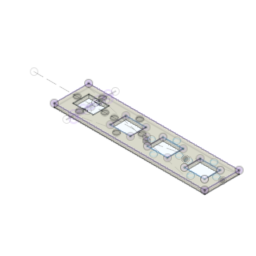
Buttons_Final (Autodesk Fusion 360 design; units mm, degrees)
Autodesk Fusion 360 part; units mm, degrees
note: some values were not read from the file. Chosen so that the rebuilt part matches the saved one: which face or edge a step refers to. Set by a fixed rule: which sketch regions a step uses.
(part 1 of 4)
sketch "Sketch1" plane through (0, 0, 0) normal (0, 1, 0) x (1, 0, 0) in component "Box"
  line L0 (86.75, -29) -> (-86.75, -29)
  line L1 (-86.75, -29) -> (-86.75, 29)
  line L2 (-86.75, 29) -> (86.75, 29)
  line L3 (86.75, 29) -> (86.75, -29)
  line L4 (86.75, -29) -> (-86.75, 29) construction
  line L5 (-86.75, -29) -> (86.75, 29) construction
  dimension "d407" = 173.5
  dimension "d408" = 58
  dimension "d1076" = 0
  dimension "d1077" = 0
  dimension "d1078" = 0
  dimension "d1079" = 0
  dimension "d1179" = 0
  dimension "d1180" = 0
  dimension "d1181" = 0
  dimension "d1182" = 0
  dimension "d1239" = 0
  dimension "d1240" = 0
  dimension "d1241" = 0
  dimension "d1242" = 0
  dimension "d1263" = 0
  dimension "d1264" = 0
  dimension "d1265" = 0
  dimension "d1266" = 0
  dimension "d1515" = 0
  dimension "d1516" = 0
  dimension "d1517" = 0
  dimension "d1518" = 0
  constraint perpendicular L0 L1
  constraint parallel L0 L2
  constraint parallel L1 L3
  constraint horizontal L0
  constraint coincident L4 origin
  constraint coincident L5 origin
  measures "d407" distance of L1.end L2.end
  measures "d408" distance of L0.end L1.end
extrude "Extrude1" add sketch "Sketch1" along normal blind 33 makes body 1 in component "Box"
sketch "Sketch2" plane through (0, 33, 0) normal (0, 1, 0) x (-1, 0, 0) in component "Box"
  line L0 (-86.75, -29) -> (86.75, -29)
  line L1 (86.75, -29) -> (86.75, 29)
  line L2 (86.75, 29) -> (-86.75, 29)
  line L3 (-86.75, 29) -> (-86.75, -29)
  line L4 (83.75, 26) -> (-83.75, 26)
  line L5 (-83.75, 26) -> (-83.75, -26)
  line L6 (-83.75, -26) -> (83.75, -26)
  line L7 (83.75, -26) -> (83.75, 26)
  dimension "d569" = -3
extrude "Extrude2" cut sketch "Sketch2" against normal up to surface (30 mm away) contours L4 L5 L6 L7 bodies 1 in component "Box"
sketch "Sketch5" plane through (0, 0, 29) normal (0, 0, 1) x (1, 0, 0) in component "Box"
  line L0 (-86.75, 0) -> (86.75, 0)
  line L1 (86.75, 0) -> (86.75, 33)
  line L2 (86.75, 33) -> (-86.75, 33)
  line L3 (-86.75, 33) -> (-86.75, 0)
  line L4 (-83.75, 3) -> (83.75, 3)
  line L5 (83.75, 3) -> (83.75, 33)
  line L6 (-83.75, 33) -> (-83.75, 3)
  line L7 (-47, 33) -> (83.75, 33)
  line L8 (86.75, 23) -> (86.75, 33)
  line L9 (83.75, 33) -> (86.75, 33)
  line L10 (-86.75, 33) -> (-83.75, 33)
  dimension "d440" = 3
  dimension "d441" = 3
  dimension "d442" = 3
  dimension "d595" = 10
  constraint coincident L2 L7.start
  constraint coincident L2 L5.end
  constraint parallel L0 L4
  constraint parallel L1 L5
  constraint parallel L3 L6
  constraint coincident L2 L6.start
  constraint coincident L1.end L2.start
  constraint coincident L1 L8.start
  constraint coincident L2.end L3.start
  measures "d440" distance of L0 L4
  measures "d441" distance of L3 L6
  measures "d442" distance of L1 L5
  measures "d595" distance of L1.end L8.start
extrude "Extrude5" cut sketch "Sketch5" against normal up to surface (3 mm away) contours L2 L4 L5 L6 L7 bodies 1 in component "Box"
sketch "Sketch3" plane through (0, 0, 29) normal (0, 0, 1) x (1, 0, 0) in component "Box"
  line L0 (-86.75, 0) -> (86.75, 0)
  line L1 (86.75, 0) -> (86.75, 33)
  line L2 (-86.75, 33) -> (-86.75, 0)
  line L3 (-86.75, 33) -> (-83.75, 33)
  line L4 (73.75, 21) -> (83.75, 21)
  line L5 (73.75, 21) -> (73.75, 3)
  line L6 (73.75, 3) -> (83.75, 3)
  line L7 (83.75, 3) -> (83.75, 21)
  line L8 (86.75, 0) -> (-86.75, 0)
  line L9 (-83.75, 33) -> (83.75, 33)
  line L10 (-83.75, 21) -> (-73.75, 21)
  line L11 (-73.75, 21) -> (-73.75, 3)
  line L12 (-73.75, 3) -> (-83.75, 3)
  line L13 (-83.75, 3) -> (-83.75, 21)
  line L14 (83.75, 33) -> (83.75, 3)
  line L15 (83.75, 3) -> (-83.75, 3)
  line L16 (-83.75, 3) -> (-83.75, 33)
  line L17 (86.75, 33) -> (83.75, 33)
  line L18 (83.75, 33) -> (86.75, 33)
  point P0 (0, 16.5)
  dimension "d424" = 10
  dimension "d1313" = 3
  dimension "d1315" = 12
  dimension "d1316" = 3
  dimension "d1566" = 10
  dimension "d1568" = 12
  dimension "d1570" = 3
  dimension "d1571" = 3
  constraint perpendicular L4 L5
  constraint perpendicular L5 L6
  constraint horizontal L10
  constraint vertical L11
  constraint horizontal L12
  constraint vertical L13
  measures "d424" distance of L4.end L4.start
  measures "d1313" distance of L6 L8
  measures "d1315" distance of L4 L9
  measures "d1316" distance of L1 L7
  measures "d1566" distance of L10.start L10.end
  measures "d1568" distance of L9 L10
  measures "d1570" distance of L8 L12
  measures "d1571" distance of L2 L13
extrude "Extrude3" add sketch "Sketch3" along normal mid plane 10 from surface at -45 contours L4 L5 L6 L7 L14 L15 bodies 1 in component "Box"
mirror "Mirror1" about plane through (0, 0, 0) normal (0, 0, 1) of "Extrude3" in component "Box"
sketch "Sketch4" plane through (0, 33, 0) normal (0, 1, 0) x (-1, 0, 0) in component "Box"
  line L0 (-86.75, -29) -> (86.75, -29)
  line L1 (86.75, -29) -> (86.75, 29)
  line L2 (-83.75, 29) -> (-86.75, 29)
  line L3 (-86.75, 29) -> (-86.75, -29)
  circle A0 centre (79.75, -24.8) radius 2
  line L4 (83.75, -26) -> (-83.75, -26)
  line L5 (-83.75, -26) -> (-83.75, 29)
  circle A1 centre (79.75, 24.8) radius 2
  line L6 (86.75, 29) -> (86.75, -29)
  line L7 (86.75, 29) -> (73.75, 29)
  line L8 (73.75, 29) -> (73.75, 21)
  line L9 (73.75, 21) -> (86.75, 21)
  line L10 (86.75, 21) -> (86.75, 29)
  line L11 (86.75, -29) -> (73.75, -29)
  line L12 (73.75, -29) -> (73.75, -21)
  line L13 (73.75, -21) -> (86.75, -21)
  line L14 (86.75, -21) -> (86.75, -29)
  line L15 (86.75, 29) -> (83.75, 29)
  dimension "d431" = 4
  dimension "d581" = 4.2
  dimension "d586" = 4
  dimension "d587" = 4.2
  dimension "d933" = 0
  dimension "d934" = 0
  dimension "d935" = 0
  dimension "d933_1" = 0
  dimension "d934_1" = 0
  dimension "d935_1" = 0
  dimension "d933_2" = 0
  dimension "d934_2" = 0
  dimension "d935_2" = 0
  dimension "d1672" = 7
  dimension "d1673" = 13
  dimension "d1674" = 8
  dimension "d1675" = 8
  dimension "d1676" = 13
  dimension "d1677" = 7
  constraint horizontal L7
  constraint vertical L8
  constraint horizontal L9
  constraint vertical L10
  constraint coincident L1.end L6.start
  constraint horizontal L11
  constraint vertical L12
  constraint horizontal L13
  constraint vertical L14
  constraint coincident L0.end L1.start
  measures "d431" diameter of A0
  measures "d581" distance of L0 A0.centre
  measures "d586" diameter of A1
  measures "d587" distance of L2 A1.centre
  measures "d1672" distance of A1.centre L6
  measures "d1673" distance of L1.end L7.end
  measures "d1674" distance of L1.end L9.end
  measures "d1675" distance of L0.end L13.end
  measures "d1676" distance of L0.end L11.end
  measures "d1677" distance of A0.centre L14
extrude "Extrude4" add sketch "Sketch4" against normal up to surface (30 mm away) contours L0 L1 L6 L11 L12 L13 L14 | L1 L6 L7 L8 L9 L10 L15 | A0 L4 | A0 L4 bodies 1 in component "Box"
mirror "Mirror2" about plane through (0, 0, 0) normal (1, 0, 0) of "Extrude4" in component "Box"
sketch "Sketch7" plane through (0, 33, 0) normal (0, 1, 0) x (-1, 0, 0) in component "Box"
  circle A0 centre (79.75, -24.8) radius 2
  line L0 (73.75, -26) -> (-73.75, -26)
  line L1 (-73.75, 29) -> (-86.75, 29)
  line L2 (-86.75, 29) -> (-86.75, -29)
  line L3 (-86.75, -29) -> (86.75, -29)
  line L4 (86.75, -29) -> (86.75, 29)
  line L5 (-73.75, 29) -> (73.75, 29)
  line L6 (86.75, 29) -> (86.75, -29)
  line L7 (-83.75, -21) -> (-83.75, 21)
  line L8 (73.75, 29) -> (73.75, 21)
  line L9 (73.75, 21) -> (83.75, 21)
  line L10 (83.75, 21) -> (83.75, -21)
  line L11 (83.75, -21) -> (73.75, -21)
  line L12 (73.75, -21) -> (73.75, -26)
  line L13 (-73.75, -26) -> (-73.75, -21)
  line L14 (-73.75, -21) -> (-83.75, -21)
  line L15 (-83.75, 21) -> (-73.75, 21)
  line L16 (-73.75, 21) -> (-73.75, 29)
  line L17 (86.75, 29) -> (73.75, 29)
  circle A1 centre (-79.75, 24.8) radius 2
  line L18 (86.75, -21) -> (86.75, -29)
  point P0 (87, 25)
  point P1 (79.75, -24.8)
  dimension "d570" = 4
  dimension "d584" = 4.2
  dimension "d1679" = 7
  measures "d570" diameter of A0
  measures "d584" distance of A0.centre L3
  measures "d1679" distance of A0.centre L18
sketch "Sketch1 (2)" plane through (0, 33, 0) normal (0, 1, 0) x (-1, 0, 0) in component "Lid"
  line L0 (-73.75, 29) -> (-86.75, 29)
  line L1 (-86.75, 29) -> (-86.75, -29)
  line L2 (-86.75, -29) -> (86.75, -29)
  line L3 (86.75, -29) -> (86.75, 29)
  line L4 (73.75, -26) -> (-73.75, -26)
  line L5 (73.75, -26) -> (-73.75, -26)
  line L6 (-83.75, 11) -> (-83.75, -11)
  line L7 (-73.75, -26) -> (73.75, -26)
  line L8 (83.75, -21) -> (83.75, 21)
  line L9 (73.75, 29) -> (-73.75, 29)
  line L10 (86.75, -29) -> (93.75, -29)
  line L11 (93.75, -29) -> (93.75, 32)
  line L12 (93.75, 32) -> (-93.75, 32)
  line L13 (-93.75, 32) -> (-93.75, -29)
  line L14 (-93.75, -29) -> (86.75, -29)
  line L15 (-93.75, 29) -> (93.75, 29)
  line L16 (93.75, 29) -> (93.75, -29)
  line L17 (93.75, -29) -> (-93.75, -29)
  line L18 (-93.75, -29) -> (-93.75, 29)
  line L19 (-93.75, 29) -> (93.75, -29) construction
  line L20 (93.75, 29) -> (-93.75, -29) construction
  line L21 (-73.75, 29) -> (-73.75, 11)
  line L22 (-73.75, 11) -> (-83.75, 11)
  line L23 (-83.75, -11) -> (-73.75, -11)
  line L24 (-73.75, -11) -> (-73.75, -26)
  line L25 (-83.75, -21) -> (-83.75, 21)
  line L26 (73.75, 29) -> (73.75, 21)
  line L27 (73.75, 21) -> (83.75, 21)
  line L28 (83.75, 21) -> (83.75, -21)
  line L29 (83.75, -21) -> (73.75, -21)
  line L30 (73.75, -21) -> (73.75, -26)
  line L31 (-73.75, -26) -> (-73.75, -21)
  line L32 (-73.75, -21) -> (-83.75, -21)
  line L33 (-83.75, 21) -> (-73.75, 21)
  line L34 (-73.75, 21) -> (-73.75, 29)
  line L35 (86.75, 29) -> (73.75, 29)
  line L36 (73.75, -26) -> (73.75, -21)
  line L37 (73.75, -21) -> (83.75, -21)
  line L38 (83.75, 21) -> (73.75, 21)
  line L39 (73.75, 21) -> (73.75, 29)
  circle A0 centre (-79.75, 24.8) radius 2
  circle A1 centre (79.75, 24.8) radius 2
  dimension "d1017" = 3
  dimension "d1018" = 10
  dimension "d1020" = 187.5
  dimension "d1072" = 0
  dimension "d1073" = 0
  dimension "d1074" = 0
  dimension "d1075" = 0
  dimension "d1235" = 0
  dimension "d1236" = 0
  dimension "d1237" = 0
  dimension "d1238" = 0
  dimension "d1449" = 0
  dimension "d1450" = 0
  dimension "d1451" = 0
  dimension "d1452" = 0
  dimension "d1463" = 0
  dimension "d1464" = 0
  dimension "d1465" = 0
  dimension "d1466" = 0
  dimension "d1495" = 0
  dimension "d1496" = 0
  dimension "d1497" = 0
  dimension "d1498" = 0
  dimension "d1507" = 0
  dimension "d1508" = 0
  dimension "d1509" = 0
  dimension "d1510" = 0
  dimension "d1511" = 0
  dimension "d1512" = 0
  dimension "d1513" = 0
  dimension "d1514" = 0
  dimension "d1531" = 0
  dimension "d1532" = 0
  dimension "d1533" = 0
  dimension "d1534" = 0
  constraint coincident L2.end L3.start
  constraint perpendicular L3 L10
  constraint perpendicular L10 L11
  constraint perpendicular L11 L12
  constraint perpendicular L12 L13
  constraint perpendicular L3 L14
  constraint perpendicular L15 L16
  constraint parallel L15 L17
  constraint parallel L16 L18
  constraint horizontal L15
  constraint coincident L13 L15.start
  constraint coincident L19 origin
  constraint coincident L20 origin
  measures "d1017" distance of L9 L12
  measures "d1018" distance of L8 L11
  measures "d1020" distance of L11.end L12.end
extrude "Extrude2'" add sketch "Sketch1 (2)" along normal blind 5.25 separate body contours L0 L1 L2 L3 L4 L5 L6 L7 L8 L14 L15 L17 L21 L24 L25 L26 L27 L28 L29 L30 L31 L32 L33 L34 L35 L36 L37 L38 L39 | L4 L5 L6 L7 L8 L9 L15 L21 L22 L23 L24 L25 L26 L27 L28 L29 L30 L31 L34 L36 L37 L38 L39 | L1 L13 L14 L15 L17 L18 | L21 L22 L25 L33 | L3 L10 L11 L15 L16 L17 | L23 L24 L25 L32 | A0 | A1 makes body 2 in component "Lid"
sketch "Sketch1 (3)" plane through (0, 3, 0) normal (0, 1, 0) x (-1, 0, 0) in component "Button Base"
  line L0 (-83.5, 19.1) -> (83.5, 19.1)
  line L1 (83.5, 19.1) -> (83.5, -19.1)
  line L2 (83.5, -19.1) -> (-83.5, -19.1)
  line L3 (-83.5, -19.1) -> (-83.5, 19.1)
  line L4 (-83.5, 19.1) -> (83.5, -19.1) construction
  line L5 (83.5, 19.1) -> (-83.5, -19.1) construction
  dimension "d738" = 167
  dimension "d739" = 38.2
  dimension "d917" = 0
  dimension "d918" = 0
  dimension "d919" = 0
  dimension "d920" = 0
  dimension "d943" = 0
  dimension "d944" = 0
  dimension "d945" = 0
  dimension "d946" = 0
  dimension "d955" = 0
  dimension "d956" = 0
  dimension "d957" = 0
  dimension "d958" = 0
  dimension "d963" = 0
  dimension "d964" = 0
  dimension "d965" = 0
  dimension "d966" = 0
  dimension "d973" = 0
  dimension "d974" = 0
  dimension "d975" = 0
  dimension "d976" = 0
  dimension "d985" = 0
  dimension "d986" = 0
  dimension "d987" = 0
  dimension "d988" = 0
  dimension "d1007" = 0
  dimension "d1008" = 0
  dimension "d1009" = 0
  dimension "d1010" = 0
  dimension "d1090" = 0
  dimension "d1091" = 0
  dimension "d1092" = 0
  dimension "d1093" = 0
  dimension "d1098" = 0
  dimension "d1099" = 0
  dimension "d1100" = 0
  dimension "d1101" = 0
  dimension "d1107" = 0
  dimension "d1108" = 0
  dimension "d1109" = 0
  dimension "d1110" = 0
  dimension "d1115" = 0
  dimension "d1116" = 0
  dimension "d1117" = 0
  dimension "d1118" = 0
  dimension "d1123" = 0
  dimension "d1124" = 0
  dimension "d1125" = 0
  dimension "d1126" = 0
  dimension "d1132" = 0
  dimension "d1133" = 0
  dimension "d1134" = 0
  dimension "d1135" = 0
  dimension "d1140" = 0
  dimension "d1141" = 0
  dimension "d1142" = 0
  dimension "d1143" = 0
  dimension "d1148" = 0
  dimension "d1149" = 0
  dimension "d1150" = 0
  dimension "d1151" = 0
  dimension "d1160" = 0
  dimension "d1161" = 0
  dimension "d1162" = 0
  dimension "d1163" = 0
  dimension "d1175" = 0
  dimension "d1176" = 0
  dimension "d1177" = 0
  dimension "d1178" = 0
  dimension "d1191" = 0
  dimension "d1192" = 0
  dimension "d1193" = 0
  dimension "d1194" = 0
  dimension "d1199" = 0
  dimension "d1200" = 0
  dimension "d1201" = 0
  dimension "d1202" = 0
  dimension "d1215" = 0
  dimension "d1216" = 0
  dimension "d1217" = 0
  dimension "d1218" = 0
  dimension "d1247" = 0
  dimension "d1248" = 0
  dimension "d1249" = 0
  dimension "d1250" = 0
  dimension "d1255" = 0
  dimension "d1256" = 0
  dimension "d1257" = 0
  dimension "d1258" = 0
  dimension "d1259" = 0
  dimension "d1260" = 0
  dimension "d1261" = 0
  dimension "d1262" = 0
  dimension "d1279" = 0
  dimension "d1280" = 0
  dimension "d1281" = 0
  dimension "d1282" = 0
  dimension "d1287" = 0
  dimension "d1288" = 0
  dimension "d1289" = 0
  dimension "d1290" = 0
  constraint perpendicular L0 L1
  constraint parallel L0 L2
  constraint parallel L1 L3
  constraint horizontal L0
  constraint coincident L4 origin
  constraint coincident L5 origin
  measures "d738" distance of L1.end L2.end
  measures "d739" distance of L0.end L1.end
extrude "Extrude1'" add sketch "Sketch1 (3)" along normal blind 4 separate body makes body 3 in component "Button Base"
sketch "Sketch2 (2)" plane through (0, 7, 0) normal (0, 1, 0) x (-1, 0, 0) in component "Button Base"
  line L0 (73, -8.7) -> (50.6, -8.7)
  line L1 (50.6, -8.7) -> (50.6, 8.7)
  line L2 (50.6, 8.7) -> (73, 8.7)
  line L3 (73, 8.7) -> (73, -8.7)
  line L4 (0, 0) -> (125, 0) construction
  line L5 (9.4, -8.7) -> (9.4, 8.7)
  line L6 (31.8, -8.7) -> (9.4, -8.7)
  line L7 (31.8, 8.7) -> (31.8, -8.7)
  line L8 (9.4, 8.7) -> (31.8, 8.7)
  line L9 (-31.8, -8.7) -> (-31.8, 8.7)
  line L10 (-9.4, -8.7) -> (-31.8, -8.7)
  line L11 (-9.4, 8.7) -> (-9.4, -8.7)
  line L12 (-31.8, 8.7) -> (-9.4, 8.7)
  line L13 (-73, -8.7) -> (-73, 8.7)
  line L14 (-50.6, 8.7) -> (-50.6, -8.7)
  line L15 (-50.6, -8.7) -> (-73, -8.7)
  line L16 (-73, 8.7) -> (-50.6, 8.7)
  line L17 (-83.5, -19.1) -> (83.5, -19.1)
  line L18 (83.5, -19.1) -> (83.5, 19.1)
  line L19 (83.5, 19.1) -> (-83.5, 19.1)
  line L20 (-83.5, 19.1) -> (-83.5, -19.1)
  point P0 (-43, 0)
  point P1 (-43, 0)
  point P2 (-84, 0)
  point P3 (-84, 0)
  point P4 (-123, 0)
  point P5 (-123, 0)
  dimension "d460" = 22.4
  dimension "d461" = 17.4
  dimension "d462" = 8.7
  dimension "d684" = 22.4
  dimension "d685" = 17.4
  dimension "d686" = 18.8
  dimension "d687" = 22.4
  dimension "d688" = 17.4
  dimension "d689" = 18.8
  dimension "d690" = 22.4
  dimension "d691" = 17.4
  dimension "d692" = 18.8
  dimension "d741" = 10.5
  dimension "d742" = 9.5
  constraint horizontal L0
  constraint vertical L1
  constraint horizontal L2
  constraint vertical L3
  constraint coincident L4.start origin
  constraint horizontal L6
  constraint vertical L5
  constraint horizontal L8
  constraint vertical L7
  constraint coincident P1 P0
  constraint horizontal L10
  constraint vertical L9
  constraint horizontal L12
  constraint vertical L11
  constraint coincident P3 P2
  constraint horizontal L15
  constraint vertical L13
  constraint horizontal L16
  constraint vertical L14
  constraint coincident P5 P4
  measures "d460" distance of L0.start L0.end
  measures "d461" distance of L0.start L2.end
  measures "d462" distance of L0 L4
  measures "d684" distance of L5.start L6.start
  measures "d685" distance of L7.start L6.start
  measures "d686" distance of L1 L7
  measures "d687" distance of L10.start L9.start
  measures "d688" distance of L10.start L11.start
  measures "d689" distance of L5 L11
  measures "d690" distance of L13.start L14.end
  measures "d691" distance of L14.start L14.end
  measures "d692" distance of L9 L14
  measures "d741" distance of L3 L18
extrude "Extrude2''" cut sketch "Sketch2 (2)" against normal up to surface (4 mm away) contours L0 L1 L2 L3 | L5 L6 L7 L8 | L9 L10 L11 L12 | L13 L14 L15 L16 bodies 3 in component "Button Base"
ref_plane "WorkPlane2" through (-61.8, 5, 0) normal (1, 0, 0) x (0, 0, 1) in component "Button Base"
sketch "Sketch3 (2)" plane through (-61.8, 5, 0) normal (1, 0, 0) x (0, 0, -1) in component "Button Base"
  line L0 (4.9445, 1.9983) -> (4.9445, 1.3202) construction
  line L1 (8.857, -2) -> (16.48, -2) construction
  line L2 (27, 1.2) -> (-27, 1.2)
  line L3 (8.857, -2) -> (8.857, 0.5)
  line L4 (8.857, 0.5) -> (6.357, 0.5)
  line L5 (8.857, -2) -> (6.357, 0.5)
  line L6 (8.857, -2) -> (11.9527, -2) construction
  line L7 (-8.7, -2) -> (-8.7, 0.5)
  line L8 (-8.7, 0.5) -> (-6.2, 0.5)
  line L9 (19.1, -2) -> (-19.1, -2)
  line L10 (-8.7, -2) -> (-6.2, 0.5)
  line L11 (-8.7, -2) -> (-4.0221, -2) construction
  line L12 (-19.1, 2) -> (19.1, 2)
  line L13 (8.7, 2) -> (-8.7, 2)
  dimension "d492" = 2.5
  dimension "d494" = 0.7
  dimension "d496" = 135
  dimension "d500" = 2.5
  dimension "d503" = 8.7
  dimension "d1321" = 45
  dimension "d1560" = 1.5
  dimension "d1561" = 1.5
  constraint vertical L0
  constraint horizontal L1
  constraint perpendicular L1 L3
  constraint perpendicular L3 L4
  constraint horizontal L6
  constraint vertical L7
  constraint perpendicular L7 L8
  constraint horizontal L11
  constraint coincident L8 L10.end
  measures "d492" distance of L1.start L3.end
  measures "d494" distance of L2 L4
  measures "d496" angle of L5 L6
  measures "d500" distance of L7.start L7.end
  measures "d503" distance of origin L7
  measures "d1321" angle of L10 L11
  measures "d1560" distance of L8 L12
  measures "d1561" distance of L4 L13
extrude "Extrude3'" add sketch "Sketch3 (2)" along normal mid plane 5 bodies 3 in component "Button Base"
sketch "Sketch4 (2)" plane through (0, 7, 0) normal (0, 1, 0) x (-1, 0, 0) in component "Button Base"
  line L0 (73, 8.7) -> (73, -8.7)
  line L1 (73, -8.7) -> (50.6, -8.7)
  line L2 (50.6, -8.7) -> (50.6, 8.7)
  line L3 (50.6, 8.7) -> (73, 8.7)
  circle A0 centre (61.8, -12.9) radius 2.95
  circle A1 centre (46.4, 0) radius 2.95
  circle A2 centre (61.8, 12.9) radius 2.95
  circle A3 centre (77.2, 0) radius 2.95
  line L4 (9.4, 8.7) -> (31.8, 8.7)
  line L5 (31.8, 8.7) -> (31.8, -8.7)
  line L6 (31.8, -8.7) -> (9.4, -8.7)
  line L7 (9.4, -8.7) -> (9.4, 8.7)
  line L8 (-31.8, 8.7) -> (-9.4, 8.7)
  line L9 (-9.4, 8.7) -> (-9.4, -8.7)
  line L10 (-9.4, -8.7) -> (-31.8, -8.7)
  line L11 (-83.5, -19.1) -> (83.5, -19.1)
  line L12 (83.5, -19.1) -> (83.5, 19.1)
  line L13 (83.5, 19.1) -> (-83.5, 19.1)
  line L14 (-83.5, 19.1) -> (-83.5, -19.1)
  line L15 (-31.8, -8.7) -> (-31.8, 8.7)
  line L16 (-73, 8.7) -> (-50.6, 8.7)
  line L17 (-50.6, 8.7) -> (-50.6, -8.7)
  line L18 (-50.6, -8.7) -> (-73, -8.7)
  line L19 (-73, -8.7) -> (-73, 8.7)
  circle A4 centre (36, 0) radius 2.95
  circle A5 centre (20.6, 12.9) radius 2.95
  circle A6 centre (5.2, 0) radius 2.95
  circle A7 centre (20.6, -12.9) radius 2.95
  circle A8 centre (-36, 0) radius 2.95
  circle A9 centre (-20.6, -12.9) radius 2.95
  line L20 (-31.8, 8.7) -> (-9.4, 8.7)
  circle A10 centre (-20.6, 12.9) radius 2.95
  line L21 (-31.8, -8.7) -> (-31.8, 8.7)
  circle A11 centre (-5.2, 0) radius 2.95
  line L22 (-9.4, -8.7) -> (-31.8, -8.7)
  circle A12 centre (-61.8, -12.9) radius 2.95
  circle A13 centre (-46.4, 0) radius 2.95
  line L23 (-73, -8.7) -> (-73, 8.7)
  circle A14 centre (-61.8, 12.9) radius 2.95
  circle A15 centre (-77.2, 0) radius 2.95
  line L24 (-72.8, 8.7) -> (-50.4, 8.7)
  dimension "d506" = 5.9
  dimension "d507" = 4.2
  dimension "d509" = 4.2
  dimension "d510" = 4.2
  dimension "d517" = 11.2
  dimension "d541" = 11.2
  dimension "d542" = 8.7
  dimension "d543" = 8.7
  dimension "d743" = 4.2
  dimension "d744" = 5.9
  dimension "d745" = 4.2
  dimension "d746" = 8.7
  dimension "d747" = 4.2
  dimension "d748" = 11.2
  dimension "d749" = 11.2
  dimension "d750" = 4.2
  dimension "d751" = 4.2
  dimension "d752" = 8.7
  dimension "d761" = 5.9
  dimension "d763" = 8.7
  dimension "d764" = 4.2
  dimension "d765" = 11.2
  dimension "d766" = 11.2
  dimension "d767" = 4.2
  dimension "d768" = 4.2
  dimension "d769" = 8.7
  dimension "d770" = 4.2
  dimension "d771" = 5.9
  dimension "d774" = 11.2
  dimension "d775" = 11.2
  dimension "d777" = 4.2
  dimension "d780" = 4.2
  dimension "d781" = 4.2
  dimension "d782" = 4.2
  constraint equal A0 A3
  constraint equal A0 A1
  constraint equal A1 A2
  constraint equal A4 A7
  constraint equal A6 A7
  constraint equal A5 A6
  constraint equal A9 A11
  constraint equal A8 A9
  constraint equal A8 A10
  constraint equal A12 A13
  constraint equal A12 A15
  constraint equal A14 A15
  measures "d506" diameter of A3
  measures "d507" distance of L1 A0.centre
  measures "d509" distance of L3 A2.centre
  measures "d510" distance of L2 A1.centre
  measures "d517" distance of L0 A0.centre
  measures "d541" distance of L0 A2.centre
  measures "d542" distance of L3 A1.centre
  measures "d543" distance of L1 A3.centre
  measures "d743" distance of L0 A3.centre
  measures "d744" diameter of A4
  measures "d745" distance of L5 A4.centre
  measures "d746" distance of L6 A4.centre
  measures "d747" distance of L6 A7.centre
  measures "d748" distance of L7 A7.centre
  measures "d749" distance of L7 A5.centre
  measures "d750" distance of L4 A5.centre
  measures "d751" distance of L7 A6.centre
  measures "d752" distance of L6 A6.centre
  measures "d761" diameter of A11
  measures "d763" distance of A11.centre L22
  measures "d764" distance of A9.centre L22
  measures "d765" distance of A9.centre L21
  measures "d766" distance of A10.centre L21
  measures "d767" distance of A10.centre L20
  measures "d768" distance of A8.centre L21
  measures "d769" distance of A8.centre L22
  measures "d770" distance of L9 A11.centre
  measures "d771" diameter of A13
  measures "d774" distance of A12.centre L23
  measures "d775" distance of A14.centre L23
  measures "d777" distance of A15.centre L23
  measures "d780" distance of L17 A13.centre
  measures "d781" distance of L18 A12.centre
  measures "d782" distance of A14.centre L24
extrude "Extrude4'" [suppressed] in component "Button Base"
sketch "Sketch5 (2)" plane through (0, 7, 0) normal (0, 1, 0) x (-1, 0, 0) in component "Button Base"
  line L0 (-116.4, -19.1) -> (-116.4, 19.1)
  line L1 (-163.8456, 0) -> (33.1232, 0) construction
  circle A0 centre (36, 0) radius 2.95
  circle A1 centre (77.2, 0) radius 2.95
  circle A2 centre (61.8, -12.9) radius 2.95
  circle A3 centre (20.6, -12.9) radius 2.95
  circle A4 centre (20.6, 12.9) radius 2.95
  circle A5 centre (61.8, 12.9) radius 2.95
  circle A6 centre (46.4, 0) radius 2.95
  circle A7 centre (5.2, 0) radius 2.95
  line L2 (9.4, 8.7) -> (31.8, 8.7)
  line L3 (31.8, 8.7) -> (31.8, -8.7)
  line L4 (31.8, -8.7) -> (9.4, -8.7)
  line L5 (9.4, -8.7) -> (9.4, 8.7)
  line L6 (-31.8, 8.7) -> (-9.4, 8.7)
  line L7 (-9.4, 8.7) -> (-9.4, -8.7)
  line L8 (-9.4, -8.7) -> (-31.8, -8.7)
  line L9 (-31.8, -8.7) -> (-31.8, 8.7)
  line L10 (73, 8.7) -> (73, -8.7)
  line L11 (73, -8.7) -> (50.6, -8.7)
  line L12 (50.6, -8.7) -> (50.6, 8.7)
  line L13 (50.6, 8.7) -> (73, 8.7)
  line L14 (-73, 8.7) -> (-50.6, 8.7)
  line L15 (-50.6, 8.7) -> (-50.6, -8.7)
  line L16 (-50.6, -8.7) -> (-73, -8.7)
  line L17 (-73, -8.7) -> (-73, 8.7)
  line L18 (-83.5, -19.1) -> (83.5, -19.1)
  line L19 (83.5, -19.1) -> (83.5, 19.1)
  line L20 (83.5, 19.1) -> (-83.5, 19.1)
  line L21 (-83.5, 19.1) -> (-83.5, -19.1)
  line L22 (81.5, 17.1) -> (-81.5, 17.1)
  line L23 (-81.5, 17.1) -> (-81.5, -17.1)
  line L24 (-81.5, -17.1) -> (81.5, -17.1)
  line L25 (81.5, -17.1) -> (81.5, 17.1)
  line L26 (42.2, -17.1) -> (40.2, -17.1)
  line L27 (40.2, -17.1) -> (40.2, 17.1)
  line L28 (40.2, 17.1) -> (42.2, 17.1)
  line L29 (42.2, 17.1) -> (42.2, -17.1)
  line L30 (1, -17.1) -> (-1, -17.1)
  line L31 (-1, -17.1) -> (-1, 17.1)
  line L32 (-1, 17.1) -> (1, 17.1)
  line L33 (1, 17.1) -> (1, -17.1)
  circle A8 centre (-61.8, 12.9) radius 2.95
  circle A9 centre (-20.6, 12.9) radius 2.95
  circle A10 centre (-5.2, 0) radius 2.95
  circle A11 centre (-61.8, -12.9) radius 2.95
  circle A12 centre (-46.4, 0) radius 2.95
  circle A13 centre (-20.6, -12.9) radius 2.95
  circle A14 centre (-36, 0) radius 2.95
  circle A15 centre (-77.2, 0) radius 2.95
  line L34 (-40.2, -17.1) -> (-42.2, -17.1)
  line L35 (-42.2, -17.1) -> (-42.2, 17.1)
  line L36 (-42.2, 17.1) -> (-40.2, 17.1)
  line L37 (-40.2, 17.1) -> (-40.2, -17.1)
  line L38 (-75.5, -19.1) -> (-83.5, -19.1)
  line L39 (-83.5, -19.1) -> (-83.5, -11.1)
  line L40 (-83.5, -11.1) -> (-75.5, -11.1)
  line L41 (-75.5, -11.1) -> (-75.5, -19.1)
  line L42 (-83.5, 19.1) -> (-75.5, 19.1)
  line L43 (-75.5, 19.1) -> (-75.5, 11.1)
  line L44 (-75.5, 11.1) -> (-83.5, 11.1)
  line L45 (-83.5, 11.1) -> (-83.5, 19.1)
  line L46 (83.5, -19.1) -> (75.5, -19.1)
  line L47 (75.5, -19.1) -> (75.5, -11.1)
  line L48 (75.5, -11.1) -> (83.5, -11.1)
  line L49 (83.5, -11.1) -> (83.5, -19.1)
  line L50 (83.5, 19.1) -> (75.5, 19.1)
  line L51 (75.5, 19.1) -> (75.5, 11.1)
  line L52 (75.5, 11.1) -> (83.5, 11.1)
  line L53 (83.5, 11.1) -> (83.5, 19.1)
  line L54 (45.2, -11.1) -> (37.2, -11.1)
  line L55 (37.2, -11.1) -> (37.2, -19.1)
  line L56 (37.2, -19.1) -> (45.2, -19.1)
  line L57 (45.2, -19.1) -> (45.2, -11.1)
  line L58 (45.2, -11.1) -> (37.2, -19.1) construction
  line L59 (37.2, -11.1) -> (45.2, -19.1) construction
  line L60 (37.2, 19.1) -> (37.2, 11.1)
  line L61 (37.2, 19.1) -> (45.2, 11.1) construction
  line L62 (45.2, 19.1) -> (37.2, 19.1)
  line L63 (42.2, 10.9) -> (40.2, 10.9)
  line L64 (45.2, 11.1) -> (45.2, 19.1)
  line L65 (45.2, 19.1) -> (37.2, 11.1) construction
  line L66 (37.2, 11.1) -> (45.2, 11.1)
  line L67 (4, -11.1) -> (-4, -11.1)
  line L68 (4, -11.1) -> (-4, -19.1) construction
  line L69 (-4, -19.1) -> (4, -19.1)
  line L70 (-4, -11.1) -> (-4, -19.1)
  line L71 (4, -19.1) -> (4, -11.1)
  line L72 (1.2, -17.1) -> (-0.8, -17.1)
  line L73 (-4, -11.1) -> (4, -19.1) construction
  line L74 (-37.2, -11.1) -> (-45.2, -11.1)
  line L75 (-37.2, -11.1) -> (-45.2, -19.1) construction
  line L76 (-45.2, -19.1) -> (-37.2, -19.1)
  line L77 (-45.2, -11.1) -> (-45.2, -19.1)
  line L78 (-37.2, -19.1) -> (-37.2, -11.1)
  line L79 (-39.8, -17.1) -> (-41.8, -17.1)
  line L80 (-45.2, -11.1) -> (-37.2, -19.1) construction
  line L81 (4, 19.1) -> (-4, 19.1)
  line L82 (4, 19.1) -> (-4, 11.1) construction
  line L83 (-4, 11.1) -> (4, 11.1)
  line L84 (-4, 19.1) -> (-4, 11.1)
  line L85 (4, 11.1) -> (4, 19.1)
  line L86 (-4, 19.1) -> (4, 11.1) construction
  line L87 (45.2, -11.1) -> (37.2, -11.1)
  line L88 (45.2, -11.1) -> (37.2, -19.1) construction
  line L89 (37.2, -19.1) -> (45.2, -19.1)
  line L90 (37.2, -11.1) -> (37.2, -19.1)
  line L91 (45.2, -19.1) -> (45.2, -11.1)
  line L92 (42.2, -17.1) -> (40.2, -17.1)
  line L93 (37.2, -11.1) -> (45.2, -19.1) construction
  line L94 (-37.2, 19.1) -> (-45.2, 19.1)
  line L95 (-45.2, 19.1) -> (-45.2, 11.1)
  line L96 (-45.2, 11.1) -> (-37.2, 11.1)
  line L97 (-37.2, 11.1) -> (-37.2, 19.1)
  line L98 (-37.2, 19.1) -> (-45.2, 11.1) construction
  line L99 (-45.2, 19.1) -> (-37.2, 11.1) construction
  point P0 (-163.8456, 0)
  point P1 (-138, 0)
  point P2 (-138.1, 12.9)
  point P3 (-162.2896, 0)
  point P4 (-138.1, -12.9)
  point P5 (-122.7, 0)
  point P6 (-110.2896, 0)
  point P7 (41.2, -15.1)
  point P8 (41.2, 15.1)
  point P9 (0, -15.1)
  point P10 (-41.2, -15.1)
  point P11 (0, 15.1)
  point P12 (41.2, -15.1)
  point P13 (-41.2, 15.1)
  dimension "d754" = 2
  dimension "d755" = 4.2
  dimension "d756" = 4.2
  dimension "d757" = 5.2
  dimension "d758" = 2
  dimension "d760" = 4.2
  dimension "d783" = 2
  dimension "d784" = 4.2
  dimension "d809" = 8
  dimension "d810" = 8
  dimension "d811" = 8
  dimension "d812" = 8
  dimension "d813" = 8
  dimension "d814" = 8
  dimension "d815" = 8
  dimension "d816" = 8
  dimension "d817" = 8
  dimension "d818" = 8
  dimension "d819" = 4
  dimension "d820" = 1
  dimension "d821" = 8
  dimension "d822" = 8
  dimension "d823" = 4
  dimension "d824" = 1
  dimension "d825" = 8
  dimension "d826" = 8
  dimension "d827" = 8
  dimension "d828" = 8
  dimension "d829" = 8
  dimension "d830" = 8
  dimension "d831" = 8
  dimension "d832" = 8
  dimension "d834" = 8
  dimension "d835" = 1
  dimension "d836" = 1
  dimension "d837" = 8
  dimension "d838" = 1
  dimension "d839" = 8
  dimension "d840" = 8
  dimension "d841" = 8
  dimension "d842" = 1
  dimension "d843" = 8
  constraint coincident P0 L1.start
  constraint horizontal L26
  constraint vertical L27
  constraint horizontal L28
  constraint vertical L29
  constraint coincident L22 L27.end
  constraint coincident L24 L26.start
  constraint horizontal L30
  constraint vertical L31
  constraint horizontal L32
  constraint vertical L33
  constraint coincident L22 L31.end
  constraint parallel L20 L22
  constraint parallel L21 L23
  constraint parallel L18 L24
  constraint parallel L19 L25
  constraint horizontal L34
  constraint vertical L35
  constraint horizontal L36
  constraint vertical L37
  constraint coincident L24 L34.start
  constraint horizontal L38
  constraint vertical L39
  constraint horizontal L40
  constraint vertical L41
  constraint coincident L21 L39.end
  constraint coincident L18 L38.start
  constraint horizontal L42
  constraint vertical L43
  constraint horizontal L44
  constraint vertical L45
  constraint coincident L20.end L21.start
  constraint horizontal L46
  constraint vertical L47
  constraint horizontal L48
  constraint vertical L49
  constraint coincident L18.end L19.start
  constraint horizontal L50
  constraint vertical L51
  constraint horizontal L52
  constraint vertical L53
  constraint coincident L19.end L20.start
  constraint perpendicular L54 L55
  constraint parallel L54 L56
  constraint parallel L55 L57
  constraint horizontal L54
  constraint coincident L58 P12
  constraint coincident L59 P12
  constraint horizontal L63
  constraint perpendicular L60 L62
  constraint parallel L62 L66
  constraint parallel L60 L64
  constraint horizontal L62
  constraint coincident P8 L65
  constraint coincident P8 L61
  constraint horizontal L72
  constraint perpendicular L67 L70
  constraint parallel L67 L69
  constraint parallel L70 L71
  constraint horizontal L67
  constraint coincident P9 L68
  constraint coincident P9 L73
  constraint horizontal L79
  constraint perpendicular L74 L77
  constraint parallel L74 L76
  constraint parallel L77 L78
  constraint horizontal L74
  constraint coincident P10 L75
  constraint coincident P10 L80
  constraint perpendicular L81 L84
  constraint parallel L81 L83
  constraint parallel L84 L85
  constraint horizontal L81
  constraint coincident P11 L82
  constraint coincident P11 L86
  constraint horizontal L92
  constraint perpendicular L87 L90
  constraint parallel L87 L89
  constraint parallel L90 L91
  constraint horizontal L87
  constraint coincident P12 L88
  constraint coincident P12 L93
  constraint perpendicular L94 L95
  constraint parallel L94 L96
  constraint parallel L95 L97
  constraint horizontal L94
  constraint coincident L98 P13
  constraint coincident L99 P13
  measures "d754" distance of L27.end L28.end
  measures "d755" distance of A0.centre L27
  measures "d756" distance of A6.centre L29
  measures "d758" distance of L31.end L32.end
  measures "d760" distance of A7.centre L33
  measures "d783" distance of L34.start L34.end
  measures "d784" distance of A14.centre L37
  measures "d809" distance of L38.start L18.start
  measures "d810" distance of L38.start L40.end
  measures "d811" distance of L20.end L44.end
  measures "d812" distance of L20.end L42.end
  measures "d813" distance of L18.end L46.end
  measures "d814" distance of L18.end L48.end
  measures "d815" distance of L19.end L50.end
  measures "d816" distance of L19.end L52.end
  measures "d817" distance of L55.end L56.end
  measures "d818" distance of L54.end L55.end
  measures "d819" distance of L18 P12
  measures "d820" distance of L27 P12
  measures "d821" distance of L61.end L60.end
  measures "d822" distance of L60.start L60.end
  measures "d823" distance of L20 P8
  measures "d824" distance of L27 P8
  measures "d825" distance of L69.end L68.end
  measures "d826" distance of L67.end L68.end
  measures "d827" distance of L76.end L75.end
  measures "d828" distance of L74.end L75.end
  measures "d829" distance of L83.end L82.end
  measures "d830" distance of L81.end L82.end
  measures "d831" distance of L56.end L55.end
  measures "d832" distance of L54.end L55.end
  measures "d834" distance of L20 L83
  measures "d835" distance of L31 P11
  measures "d836" distance of L35 P10
  measures "d837" distance of L18 L74
  measures "d838" distance of L31 P9
  measures "d839" distance of L18 L67
  measures "d840" distance of L95.end L96.end
  measures "d841" distance of L94.end L95.end
  measures "d842" distance of L35 P13
  measures "d843" distance of L20 L96
extrude "Extrude5'" [suppressed] in component "Button Base"
sketch "Sketch6" plane through (0, 7, 0) normal (0, 1, 0) x (-1, 0, 0) in component "Button Base"
extrude "Extrude9" [suppressed] in component "Box"
thread "Thread1" [suppressed] in component "Box"
mirror "Mirror4" [suppressed] in component "Box"
sketch "Sketch1 (4)" plane through (0, 45, 0) normal (0, 1, 0) x (-1, 0, 0) in component "Button"
  line L0 (-111.8498, 7.1011) -> (-111.8498, -10.2989)
  line L1 (-111.8498, -10.2989) -> (-134.2498, -10.2989)
  line L2 (-134.2498, -10.2989) -> (-134.2498, 7.1011)
  line L3 (-134.2498, 7.1011) -> (-111.8498, 7.1011)
  circle A0 centre (-138.4498, -1.5989) radius 3.1
  circle A1 centre (-123.0498, 11.3011) radius 3.1
  circle A2 centre (-123.0498, -14.4989) radius 3.1
  circle A3 centre (-107.6498, -1.5989) radius 3.1
  line L4 (-103.4498, -18.6989) -> (-103.4498, 15.5011)
  line L5 (-103.4498, 15.5011) -> (-142.6498, 15.5011)
  line L6 (-142.6498, 15.5011) -> (-142.6498, -18.6989)
  line L7 (-142.6498, -18.6989) -> (-103.4498, -18.6989)
  circle A4 centre (-138.4498, -1.5989) radius 3.1
  circle A5 centre (-123.0498, -14.4989) radius 3.1
  circle A6 centre (-107.6498, -1.5989) radius 3.1
  circle A7 centre (-123.0498, 11.3011) radius 3.1
  line L8 (-154.8498, 7.1011) -> (-154.8498, -10.2989)
  line L9 (-177.2498, -10.2989) -> (-177.2498, 7.1011)
  line L10 (-146.7095, 15.4507) -> (-185.4095, 15.5014)
  line L11 (-177.2498, 7.1011) -> (-154.8498, 7.1011)
  circle A8 centre (-166.0498, -14.4989) radius 3.1
  circle A9 centre (-181.4498, -1.5989) radius 3.1
  line L12 (-185.4095, 15.5014) -> (-185.4536, -18.1986)
  circle A10 centre (-181.4498, -1.5989) radius 3.1
  line L13 (-146.7537, -18.2493) -> (-146.7095, 15.4507)
  circle A11 centre (-166.0498, 11.3011) radius 3.1
  circle A12 centre (-166.0498, 11.3011) radius 3.1
  line L14 (-154.8498, -10.2989) -> (-177.2498, -10.2989)
  circle A13 centre (-150.6498, -1.5989) radius 3.1
  circle A14 centre (-150.6498, -1.5989) radius 3.1
  line L15 (-185.4536, -18.1986) -> (-146.7537, -18.2493)
  circle A15 centre (-166.0498, -14.4989) radius 3.1
  arc A16 (86.5, -27.2432) -> (86.5, -22.3568) centre (88.5, -24.8) ccw
  arc A17 (-86.5, -22.3568) -> (-86.5, -27.2432) centre (-88.5, -24.8) ccw
  line L16 (86.5, 29) -> (-86.5, 29)
  line L17 (-86.5, 29) -> (-86.5, 27.2432)
  line L18 (-86.5, -29) -> (86.5, -29)
  line L19 (86.5, -29) -> (86.5, -27.2432)
  arc A18 (86.5, 22.3568) -> (86.5, 27.2432) centre (88.5, 24.8) ccw
  arc A19 (-86.5, 27.2432) -> (-86.5, 22.3568) centre (-88.5, 24.8) ccw
  line L20 (-86.5, 22.3568) -> (-86.5, -22.3568)
  line L21 (-86.5, -27.2432) -> (-86.5, -29)
  line L22 (86.5, -22.3568) -> (86.5, 22.3568)
  line L23 (86.5, 27.2432) -> (86.5, 29)
  dimension "d623" = 39.2
  dimension "d624" = 38.7
  dimension "d625" = 33.7
  dimension "d921" = 0
  dimension "d922" = 0
  dimension "d923" = 0
  dimension "d924" = 0
  dimension "d1144" = 0
  dimension "d1145" = 0
  dimension "d1146" = 0
  dimension "d1147" = 0
  dimension "d1156" = 0
  dimension "d1157" = 0
  dimension "d1158" = 0
  dimension "d1159" = 0
  dimension "d1187" = 0
  dimension "d1188" = 0
  dimension "d1189" = 0
  dimension "d1190" = 0
  dimension "d1195" = 0
  dimension "d1196" = 0
  dimension "d1197" = 0
  dimension "d1198" = 0
  dimension "d1391" = 0
  dimension "d1392" = 0
  dimension "d1393" = 0
  dimension "d1394" = 0
  dimension "d1403" = 0
  dimension "d1404" = 0
  dimension "d1405" = 0
  dimension "d1406" = 0
  dimension "d1413" = 0
  dimension "d1414" = 0
  dimension "d1415" = 0
  dimension "d1416" = 0
  dimension "d1421" = 0
  dimension "d1422" = 0
  dimension "d1423" = 0
  dimension "d1424" = 0
  dimension "d1429" = 0
  dimension "d1430" = 0
  dimension "d1431" = 0
  dimension "d1432" = 0
  dimension "d1445" = 0
  dimension "d1446" = 0
  dimension "d1447" = 0
  dimension "d1448" = 0
  dimension "d1459" = 0
  dimension "d1460" = 0
  dimension "d1461" = 0
  dimension "d1462" = 0
  dimension "d1491" = 0
  dimension "d1492" = 0
  dimension "d1493" = 0
  dimension "d1494" = 0
  dimension "d1503" = 0
  dimension "d1504" = 0
  dimension "d1505" = 0
  dimension "d1506" = 0
  dimension "d1527" = 0
  dimension "d1528" = 0
  dimension "d1529" = 0
  dimension "d1530" = 0
  constraint perpendicular L12 L15
  constraint parallel L10 L15
  constraint parallel L12 L13
  measures "d623" distance of L4.start L6.end
  measures "d624" distance of L13.start L12.end
  measures "d625" vertical distance of L10.end L12.end
extrude "Extrude1''" [suppressed] in component "Button"
sketch "Sketch2 (3)" plane through (0, 45, 0) normal (0, 1, 0) x (-1, 0, 0) in component "Button"
  line L0 (-142.6498, -18.6989) -> (-103.4498, -18.6989)
  line L1 (-103.4498, -18.6989) -> (-103.4498, 15.5011)
  line L2 (-103.4498, 15.5011) -> (-142.6498, 15.5011)
  line L3 (-142.6498, 15.5011) -> (-142.6498, -18.6989)
extrude "Extrude2'''" [suppressed] in component "Button"
sketch "Sketch3 (3)" plane through (0, 49.8, 0) normal (0, 1, 0) x (-1, 0, 0) in component "Button"
  line L0 (-142.6498, 15.5011) -> (-142.6498, -18.6989)
  line L1 (-142.6498, -18.6989) -> (-103.4498, -18.6989)
  line L2 (-103.4498, -18.6989) -> (-103.4498, 15.5011)
  line L3 (-103.4498, 15.5011) -> (-142.6498, 15.5011)
  circle A0 centre (-123.0498, -1.5989) radius 14
  dimension "d616" = 28
  dimension "d617" = 17.1
  dimension "d618" = 34.2
  dimension "d619" = 39.2
  dimension "d620" = 19.6
  measures "d616" diameter of A0
  measures "d617" distance of L1 A0.centre
  measures "d618" distance of L1 L3
  measures "d619" distance of L0 L2
  measures "d620" distance of L2 A0.centre
extrude "Extrude3''" [suppressed] in component "Button"
sketch "Sketch4 (3)" plane through (0, 49.8, 0) normal (0, 1, 0) x (-1, 0, 0) in component "Button"
  circle A0 centre (-123.0498, -1.5989) radius 14
  line L0 (-142.6498, 15.5011) -> (-142.6498, -18.6989)
  line L1 (-142.6498, -18.6989) -> (-103.4498, -18.6989)
  line L2 (-103.4498, -18.6989) -> (-103.4498, 15.5011)
  line L3 (-103.4498, 15.5011) -> (-142.6498, 15.5011)
  line L4 (-103.9498, 15.0011) -> (-142.1498, 15.0011)
  line L5 (-142.1498, 15.0011) -> (-142.1498, -18.1989)
  line L6 (-142.1498, -18.1989) -> (-103.9498, -18.1989)
  line L7 (-103.9498, -18.1989) -> (-103.9498, 15.0011)
  dimension "d627" = -0.5
extrude "Extrude4''" [suppressed] in component "Button"
pattern_linear "R-Pattern4" [suppressed] in component "Button Base"
sketch "Sketch12" plane through (0, 7, 0) normal (0, 1, 0) x (-1, 0, 0) in component "Button Base"
  line L0 (75.5, 17.1) -> (45.2, 17.1)
  line L1 (-81.5, 11.1) -> (-81.5, -11.1)
  line L2 (-75.5, -17.1) -> (-45.2, -17.1)
  line L3 (-42.2, -11.1) -> (-42.2, 11.1)
  circle A0 centre (-61.8, 12.9) radius 2.95
  circle A1 centre (-61.8, -12.9) radius 2.95
  circle A2 centre (-46.4, 0) radius 2.95
  circle A3 centre (-77.2, 0) radius 2.95
  line L4 (-73, 8.7) -> (-50.6, 8.7)
  line L5 (-50.6, 8.7) -> (-50.6, -8.7)
  line L6 (-50.6, -8.7) -> (-73, -8.7)
  line L7 (-73, -8.7) -> (-73, 8.7)
  circle A4 centre (-79.5, -15.1) radius 3.05
  circle A5 centre (-79.5, 15.1) radius 3.05
  line L8 (-83.5, 11.1) -> (-83.5, -11.1)
  line L9 (-81.5, -11.1) -> (-83.5, -11.1)
  line L10 (-83.5, -11.1) -> (-83.5, -19.1)
  line L11 (-83.5, -19.1) -> (-75.5, -19.1)
  line L12 (-75.5, -19.1) -> (-75.5, -17.1)
  line L13 (-75.5, 17.1) -> (-75.5, 19.1)
  line L14 (83.5, 19.1) -> (75.5, 19.1)
  line L15 (-83.5, 19.1) -> (-83.5, 11.1)
  line L16 (-83.5, 11.1) -> (-81.5, 11.1)
  line L17 (-45.2, -17.1) -> (-45.2, -19.1)
  line L18 (-45.2, -19.1) -> (-37.2, -19.1)
  line L19 (-37.2, -19.1) -> (-37.2, -17.1)
  line L20 (-37.2, -17.1) -> (-4, -17.1)
  line L21 (-4, -17.1) -> (-4, -19.1)
  line L22 (-4, -19.1) -> (4, -19.1)
  line L23 (4, -19.1) -> (4, -17.1)
  line L24 (4, -17.1) -> (37.2, -17.1)
  line L25 (37.2, -17.1) -> (37.2, -19.1)
  line L26 (37.2, -19.1) -> (45.2, -19.1)
  line L27 (45.2, -19.1) -> (45.2, -17.1)
  line L28 (45.2, -17.1) -> (75.5, -17.1)
  line L29 (75.5, -17.1) -> (75.5, -19.1)
  line L30 (75.5, -19.1) -> (83.5, -19.1)
  line L31 (83.5, -19.1) -> (83.5, -11.1)
  line L32 (83.5, -11.1) -> (81.5, -11.1)
  line L33 (81.5, -11.1) -> (81.5, 11.1)
  line L34 (81.5, 11.1) -> (83.5, 11.1)
  line L35 (83.5, 11.1) -> (83.5, 19.1)
  line L36 (75.5, 19.1) -> (75.5, 17.1)
  line L37 (45.2, 17.1) -> (45.2, 19.1)
  line L38 (45.2, 19.1) -> (37.2, 19.1)
  line L39 (37.2, 19.1) -> (37.2, 17.1)
  line L40 (37.2, 17.1) -> (4, 17.1)
  line L41 (4, 17.1) -> (4, 19.1)
  line L42 (4, 19.1) -> (-4, 19.1)
  line L43 (-4, 19.1) -> (-4, 17.1)
  line L44 (-4, 17.1) -> (-37.2, 17.1)
  line L45 (-37.2, 17.1) -> (-37.2, 19.1)
  line L46 (-37.2, 19.1) -> (-45.2, 19.1)
  line L47 (-45.2, 19.1) -> (-45.2, 17.1)
  line L48 (-45.2, 17.1) -> (-75.5, 17.1)
  line L49 (-1, -11.1) -> (-1, 11.1)
  line L50 (-1, 11.1) -> (1, 11.1)
  line L51 (1, 11.1) -> (1, -11.1)
  line L52 (1, -11.1) -> (-1, -11.1)
  line L53 (-42.2, 11.1) -> (-40.2, 11.1)
  line L54 (-40.2, 11.1) -> (-40.2, -11.1)
  line L55 (-40.2, -11.1) -> (-42.2, -11.1)
  circle A6 centre (-20.6, 12.9) radius 2.95
  circle A7 centre (36, 0) radius 2.95
  circle A8 centre (77.2, 0) radius 2.95
  circle A9 centre (61.8, -12.9) radius 2.95
  circle A10 centre (20.6, -12.9) radius 2.95
  circle A11 centre (-5.2, 0) radius 2.95
  circle A12 centre (-20.6, -12.9) radius 2.95
  circle A13 centre (20.6, 12.9) radius 2.95
  circle A14 centre (61.8, 12.9) radius 2.95
  circle A15 centre (46.4, 0) radius 2.95
  circle A16 centre (5.2, 0) radius 2.95
  circle A17 centre (-36, 0) radius 2.95
  line L56 (9.4, 8.7) -> (31.8, 8.7)
  line L57 (31.8, 8.7) -> (31.8, -8.7)
  line L58 (31.8, -8.7) -> (9.4, -8.7)
  line L59 (9.4, -8.7) -> (9.4, 8.7)
  line L60 (-31.8, 8.7) -> (-9.4, 8.7)
  line L61 (-9.4, 8.7) -> (-9.4, -8.7)
  line L62 (-9.4, -8.7) -> (-31.8, -8.7)
  line L63 (-31.8, -8.7) -> (-31.8, 8.7)
  line L64 (73, 8.7) -> (73, -8.7)
  line L65 (73, -8.7) -> (50.6, -8.7)
  line L66 (50.6, -8.7) -> (50.6, 8.7)
  line L67 (50.6, 8.7) -> (73, 8.7)
  line L68 (42.2, 11.1) -> (42.2, -11.1)
  line L69 (42.2, -11.1) -> (40.2, -11.1)
  line L70 (40.2, -11.1) -> (40.2, 11.1)
  line L71 (40.2, 11.1) -> (42.2, 11.1)
  line L72 (-75.5, -19.1) -> (-45.2, -19.1)
  line L73 (4, -19.1) -> (37.2, -19.1)
  line L74 (45.2, -19.1) -> (75.5, -19.1)
  line L75 (-45.2, 19.1) -> (-75.5, 19.1)
  line L76 (75.5, 19.1) -> (45.2, 19.1)
  line L77 (-4, 19.1) -> (-37.2, 19.1)
  line L78 (-37.2, -19.1) -> (-4, -19.1)
  line L79 (37.2, 19.1) -> (4, 19.1)
  line L80 (-75.5, 19.1) -> (-83.5, 19.1)
  line L81 (-83.5, 19.1) -> (-75.5, 19.1)
  line L82 (-75.5, -19.1) -> (-83.5, -19.1)
  dimension "d790" = 4
  dimension "d791" = 6.1
  dimension "d792" = 6.1
  dimension "d793" = 4
  dimension "d1562" = 4
  dimension "d1563" = 4
  measures "d790" distance of A5.centre L8
  measures "d791" diameter of A5
  measures "d792" diameter of A4
  measures "d793" distance of A4.centre L8
  measures "d1562" distance of A5.centre L81
  measures "d1563" distance of A4.centre L82
extrude "Extrude8" [suppressed] in component "Button Base"